snek (Autodesk Fusion 360 design; units mm, degrees)
Autodesk Fusion 360 part; units mm, degrees
sketch "Sketch1" plane through (0, 0, 0) normal (0, 1, 0) x (1, 0, 0)
  spline S0 degree 3 poles (29.3103, -75.7968) (29.3103, -75.278) (29.4828, -74.6533) (29.8072, -73.9977) knots 0 0 0 0 1 1 1 1
  spline S1 degree 3 poles (29.8072, -73.9977) (30.0802, -73.4455) (30.4104, -72.7171) (30.5406, -72.3792) knots 0 0 0 0 1 1 1 1
  spline S2 degree 3 poles (30.5406, -72.3792) (30.9121, -71.4166) (34.8067, -66.1972) (35.4505, -65.7995) knots 0 0 0 0 1 1 1 1
  spline S3 degree 3 poles (35.4505, -65.7995) (35.918, -65.5106) (35.5103, -65.1333) (33.9175, -64.3814) knots 0 0 0 0 1 1 1 1
  spline S4 degree 3 poles (33.9175, -64.3814) (30.1151, -62.5864) (30.475, -62.841) (26.8195, -59.3612) knots 0 0 0 0 1 1 1 1
  spline S5 degree 3 poles (26.8195, -59.3612) (25.1375, -57.7599) (29.2799, -57.0601) (33.624, -58.2115) knots 0 0 0 0 1 1 1 1
  spline S6 degree 3 poles (33.624, -58.2115) (37.4637, -59.2291) (41.6224, -60.9553) (44.4921, -62.7222) knots 0 0 0 0 1 1 1 1
  line L0 (44.4921, -62.7222) -> (45.7208, -63.4786)
  line L1 (45.7208, -63.4786) -> (49.1432, -63.3633)
  spline S7 degree 3 poles (49.1432, -63.3633) (58.6515, -63.0423) (60.9023, -62.6732) (60.9023, -61.435) knots 0 0 0 0 1 1 1 1
  spline S8 degree 3 poles (60.9023, -61.435) (60.9023, -60.7743) (57.5045, -58.9706) (53.1077, -57.2969) knots 0 0 0 0 1 1 1 1
  spline S9 degree 3 poles (53.1077, -57.2969) (51.2821, -56.6021) (48.1624, -55.3189) (46.1751, -54.4455) knots 0 0 0 0 1 1 1 1
  spline S10 degree 3 poles (46.1751, -54.4455) (44.1875, -53.5721) (41.6243, -52.5132) (40.4789, -52.0925) knots 0 0 0 0 1 1 1 1
  spline S11 degree 3 poles (40.4789, -52.0925) (37.0141, -50.8199) (36.5223, -50.4214) (34.6461, -47.3689) knots 0 0 0 0 1 1 1 1
  spline S12 degree 3 poles (34.6461, -47.3689) (33.9934, -46.3072) (33.0015, -44.694) (32.4419, -43.7841) knots 0 0 0 0 1 1 1 1
  spline S13 degree 3 poles (32.4419, -43.7841) (30.8578, -41.2086) (30.8017, -40.965) (30.8052, -36.6557) knots 0 0 0 0 1 1 1 1
  line L2 (30.8052, -36.6557) -> (30.8083, -32.9629)
  line L3 (30.8083, -32.9629) -> (31.595, -31.573)
  spline S14 degree 3 poles (31.595, -31.573) (34.8697, -25.789) (41.12, -23.876) (55.3739, -24.2957) knots 0 0 0 0 1 1 1 1
  spline S15 degree 3 poles (55.3739, -24.2957) (62.7089, -24.5116) (63.6588, -24.6338) (67.6595, -25.8789) knots 0 0 0 0 1 1 1 1
  spline S16 degree 3 poles (67.6595, -25.8789) (68.2387, -26.0591) (70.9941, -26.9198) (73.7822, -27.7916) knots 0 0 0 0 1 1 1 1
  spline S17 degree 3 poles (73.7822, -27.7916) (78.3857, -29.2307) (78.9387, -29.3664) (79.7965, -29.2656) knots 0 0 0 0 1 1 1 1
  spline S18 degree 3 poles (79.7965, -29.2656) (81.5671, -29.0574) (82.6505, -30.8647) (81.1967, -31.6006) knots 0 0 0 0 1 1 1 1
  spline S19 degree 3 poles (81.1967, -31.6006) (80.2539, -32.0776) (80.0513, -32.339) (80.1505, -32.9502) knots 0 0 0 0 1 1 1 1
  spline S20 degree 3 poles (80.1505, -32.9502) (80.3079, -33.9194) (79.8743, -34.1249) (77.1004, -34.3969) knots 0 0 0 0 1 1 1 1
  spline S21 degree 3 poles (77.1004, -34.3969) (75.7693, -34.5274) (74.1667, -34.7187) (73.5394, -34.8216) knots 0 0 0 0 1 1 1 1
  spline S22 degree 3 poles (73.5394, -34.8216) (72.1064, -35.0568) (68.358, -34.6904) (64.6139, -33.949) knots 0 0 0 0 1 1 1 1
  spline S23 degree 3 poles (64.6139, -33.949) (55.5281, -32.1498) (47.0855, -31.9747) (44.4304, -33.5304) knots 0 0 0 0 1 1 1 1
  spline S24 degree 3 poles (44.4304, -33.5304) (41.8722, -35.0293) (40.5109, -38.4289) (41.2446, -41.4867) knots 0 0 0 0 1 1 1 1
  spline S25 degree 3 poles (41.2446, -41.4867) (41.8722, -44.1029) (47.5835, -46.9927) (55.1236, -48.509) knots 0 0 0 0 1 1 1 1
  spline S26 degree 3 poles (55.1236, -48.509) (62.1797, -49.928) (66.012, -51.9758) (68.9787, -55.9129) knots 0 0 0 0 1 1 1 1
  spline S27 degree 3 poles (68.9787, -55.9129) (71.8979, -59.7871) (72.8025, -63.3955) (71.6878, -66.7184) knots 0 0 0 0 1 1 1 1
  spline S28 degree 3 poles (71.6878, -66.7184) (69.8733, -72.1265) (67.651, -73.1063) (58.0943, -72.7105) knots 0 0 0 0 1 1 1 1
  spline S29 degree 3 poles (58.0943, -72.7105) (54.8606, -72.5766) (50.7534, -72.4631) (48.9678, -72.4583) knots 0 0 0 0 1 1 1 1
  spline S30 degree 3 poles (48.9678, -72.4583) (46.7426, -72.4522) (45.5549, -72.3789) (45.1943, -72.2252) knots 0 0 0 0 1 1 1 1
  spline S31 degree 3 poles (45.1943, -72.2252) (44.5603, -71.9553) (41.6888, -71.3328) (41.0602, -71.3291) knots 0 0 0 0 1 1 1 1
  spline S32 degree 3 poles (41.0602, -71.3291) (40.5273, -71.3256) (39.7507, -72.0924) (39.0493, -73.3145) knots 0 0 0 0 1 1 1 1
  spline S33 degree 3 poles (39.0493, -73.3145) (37.8719, -75.3658) (36.8498, -75.8725) (36.1553, -74.7488) knots 0 0 0 0 1 1 1 1
  spline S34 degree 3 poles (36.1553, -74.7488) (35.6719, -73.9667) (35.8632, -73.9278) (33.1203, -75.3629) knots 0 0 0 0 1 1 1 1
  spline S35 degree 3 poles (33.1203, -75.3629) (31.3074, -76.3114) (30.6057, -76.5916) (30.0413, -76.5916) knots 0 0 0 0 1 1 1 1
  line L4 (30.0413, -76.5916) -> (29.3103, -76.5916)
  line L5 (29.3103, -76.5916) -> (29.3103, -75.7968)
  spline S36 degree 3 poles (35.8775, -71.6704) (35.9746, -71.5757) (35.9137, -71.237) (35.724, -70.8163) knots 0 0 0 0 1 1 1 1
  spline S37 degree 3 poles (35.724, -70.8163) (34.9062, -69.0028) (36.4964, -68.0477) (37.8584, -69.5344) knots 0 0 0 0 1 1 1 1
  line L6 (37.8584, -69.5344) -> (38.4207, -70.1485)
  line L7 (38.4207, -70.1485) -> (39.4496, -69.8598)
  spline S38 degree 3 poles (39.4496, -69.8598) (40.0153, -69.7011) (40.993, -69.5712) (41.6219, -69.5712) knots 0 0 0 0 1 1 1 1
  line L8 (41.6219, -69.5712) -> (42.7651, -69.5712)
  line L9 (42.7651, -69.5712) -> (43.3443, -68.765)
  spline S39 degree 3 poles (43.3443, -68.765) (44.886, -66.6179) (46.8313, -66.846) (47.0011, -69.1936) knots 0 0 0 0 1 1 1 1
  spline S40 degree 3 poles (47.0011, -69.1936) (47.0477, -69.836) (47.1596, -70.2718) (47.2776, -70.2697) knots 0 0 0 0 1 1 1 1
  spline S41 degree 3 poles (47.2776, -70.2697) (47.3866, -70.2678) (48.3312, -70.1525) (49.3765, -70.0133) knots 0 0 0 0 1 1 1 1
  spline S42 degree 3 poles (49.3765, -70.0133) (51.1482, -69.7775) (51.389, -69.7834) (52.9196, -70.0982) knots 0 0 0 0 1 1 1 1
  spline S43 degree 3 poles (52.9196, -70.0982) (58.5512, -71.2571) (65.4124, -70.9547) (67.6103, -69.4508) knots 0 0 0 0 1 1 1 1
  spline S44 degree 3 poles (67.6103, -69.4508) (69.6047, -68.0866) (70.5818, -64.2419) (69.6534, -61.4135) knots 0 0 0 0 1 1 1 1
  spline S45 degree 3 poles (69.6534, -61.4135) (69.1793, -59.97) (68.9761, -59.9623) (68.9761, -61.3884) knots 0 0 0 0 1 1 1 1
  spline S46 degree 3 poles (68.9761, -61.3884) (68.9761, -63.984) (67.8765, -63.2474) (67.5674, -60.4446) knots 0 0 0 0 1 1 1 1
  spline S47 degree 3 poles (67.5674, -60.4446) (67.1227, -56.41) (65.7439, -54.6108) (61.5167, -52.5487) knots 0 0 0 0 1 1 1 1
  spline S48 degree 3 poles (61.5167, -52.5487) (59.1042, -51.3715) (57.6249, -50.9683) (52.1269, -49.9891) knots 0 0 0 0 1 1 1 1
  spline S49 degree 3 poles (52.1269, -49.9891) (48.1394, -49.2787) (43.8092, -47.3393) (41.1242, -45.0615) knots 0 0 0 0 1 1 1 1
  spline S50 degree 3 poles (41.1242, -45.0615) (38.7247, -43.0253) (38.2204, -37.7807) (40.15, -34.9258) knots 0 0 0 0 1 1 1 1
  spline S51 degree 3 poles (40.15, -34.9258) (42.8884, -30.8745) (45.8338, -29.9183) (54.1451, -30.3821) knots 0 0 0 0 1 1 1 1
  spline S52 degree 3 poles (54.1451, -30.3821) (56.6883, -30.524) (57.2132, -30.5094) (57.6987, -30.2827) knots 0 0 0 0 1 1 1 1
  spline S53 degree 3 poles (57.6987, -30.2827) (58.2433, -30.0284) (58.3681, -30.0493) (60.507, -30.7544) knots 0 0 0 0 1 1 1 1
  spline S54 degree 3 poles (60.507, -30.7544) (65.0624, -32.2559) (68.6115, -32.6917) (73.7153, -32.3763) knots 0 0 0 0 1 1 1 1
  spline S55 degree 3 poles (73.7153, -32.3763) (79.2983, -32.0313) (79.2578, -31.6887) (73.4076, -29.7633) knots 0 0 0 0 1 1 1 1
  spline S56 degree 3 poles (73.4076, -29.7633) (64.7663, -26.9195) (60.4938, -26.2258) (51.6004, -26.2221) knots 0 0 0 0 1 1 1 1
  spline S57 degree 3 poles (51.6004, -26.2221) (42.1579, -26.2184) (35.3579, -28.4938) (33.4277, -32.3028) knots 0 0 0 0 1 1 1 1
  line L10 (33.4277, -32.3028) -> (32.9083, -33.328)
  line L11 (32.9083, -33.328) -> (32.9083, -36.7504)
  line L12 (32.9083, -36.7504) -> (32.9083, -40.1731)
  line L13 (32.9083, -40.1731) -> (33.4518, -41.3137)
  spline S58 degree 3 poles (33.4518, -41.3137) (33.7505, -41.9413) (34.4218, -43.0475) (34.9435, -43.7724) knots 0 0 0 0 1 1 1 1
  spline S59 degree 3 poles (34.9435, -43.7724) (35.4653, -44.4971) (36.1984, -45.6817) (36.5731, -46.405) knots 0 0 0 0 1 1 1 1
  spline S60 degree 3 poles (36.5731, -46.405) (37.7756, -48.7265) (38.3421, -49.135) (42.4519, -50.645) knots 0 0 0 0 1 1 1 1
  spline S61 degree 3 poles (42.4519, -50.645) (45.7589, -51.86) (48.2669, -52.8995) (49.9914, -53.77) knots 0 0 0 0 1 1 1 1
  spline S62 degree 3 poles (49.9914, -53.77) (50.7958, -54.1761) (53.0701, -55.1244) (55.0455, -55.8774) knots 0 0 0 0 1 1 1 1
  spline S63 degree 3 poles (55.0455, -55.8774) (58.5708, -57.2212) (59.5307, -57.7237) (61.3947, -59.2027) knots 0 0 0 0 1 1 1 1
  spline S64 degree 3 poles (61.3947, -59.2027) (64.5139, -61.6773) (62.9571, -64.247) (57.8625, -65.0338) knots 0 0 0 0 1 1 1 1
  spline S65 degree 3 poles (57.8625, -65.0338) (52.8259, -65.8117) (43.7023, -65.6844) (43.7023, -64.8362) knots 0 0 0 0 1 1 1 1
  spline S66 degree 3 poles (43.7023, -64.8362) (43.7023, -64.3441) (41.7303, -63.3815) (36.4577, -61.2998) knots 0 0 0 0 1 1 1 1
  spline S67 degree 3 poles (36.4577, -61.2998) (33.8217, -60.2592) (30.7144, -59.5847) (30.7144, -60.0531) knots 0 0 0 0 1 1 1 1
  spline S68 degree 3 poles (30.7144, -60.0531) (30.7144, -60.3629) (31.4399, -60.7976) (36.241, -63.3635) knots 0 0 0 0 1 1 1 1
  spline S69 degree 3 poles (36.241, -63.3635) (39.0403, -64.8597) (39.1933, -65.4757) (37.1991, -67.2246) knots 0 0 0 0 1 1 1 1
  spline S70 degree 3 poles (37.1991, -67.2246) (35.5653, -68.6576) (32.4697, -72.4226) (32.4697, -72.9769) knots 0 0 0 0 1 1 1 1
  spline S71 degree 3 poles (32.4697, -72.9769) (32.4697, -73.2227) (35.4616, -72.0757) (35.8775, -71.6704) knots 0 0 0 0 1 1 1 1
  spline S72 degree 3 poles (53.1799, -52.9781) (51.7803, -52.3428) (50.5357, -51.7795) (50.4142, -51.7266) knots 0 0 0 0 1 1 1 1
  spline S73 degree 3 poles (50.4142, -51.7266) (50.1637, -51.6173) (49.9218, -50.8318) (50.0875, -50.6662) knots 0 0 0 0 1 1 1 1
  spline S74 degree 3 poles (50.0875, -50.6662) (50.4153, -50.3383) (57.0373, -52.8074) (57.0405, -53.2588) knots 0 0 0 0 1 1 1 1
  spline S75 degree 3 poles (57.0405, -53.2588) (57.0479, -54.3134) (55.9446, -54.2333) (53.1799, -52.9781) knots 0 0 0 0 1 1 1 1
  spline S76 degree 3 poles (36.7927, -44.7416) (36.1196, -43.5909) (36.0751, -43.1486) (36.5898, -42.7215) knots 0 0 0 0 1 1 1 1
  spline S77 degree 3 poles (36.5898, -42.7215) (36.98, -42.3977) (37.4711, -42.7792) (37.9809, -43.8023) knots 0 0 0 0 1 1 1 1
  spline S78 degree 3 poles (37.9809, -43.8023) (39.0805, -46.009) (38.023, -46.8448) (36.7927, -44.7416) knots 0 0 0 0 1 1 1 1
  line L14 (36.3667, -33.7172) -> (35.9905, -33.3169)
  line L15 (35.9905, -33.3169) -> (37.1369, -31.304)
  spline S79 degree 3 poles (37.1369, -31.304) (38.8284, -28.3345) (38.7146, -28.4756) (39.2279, -28.7095) knots 0 0 0 0 1 1 1 1
  spline S80 degree 3 poles (39.2279, -28.7095) (39.842, -28.9891) (39.7925, -29.2431) (38.6853, -31.5032) knots 0 0 0 0 1 1 1 1
  spline S81 degree 3 poles (38.6853, -31.5032) (37.3351, -34.2588) (37.093, -34.4903) (36.3667, -33.7172) knots 0 0 0 0 1 1 1 1
  spline S82 degree 3 poles (59.5148, -29.577) (58.9246, -29.4117) (58.6655, -28.9582) (58.9595, -28.6039) knots 0 0 0 0 1 1 1 1
  spline S83 degree 3 poles (58.9595, -28.6039) (59.3233, -28.1657) (61.277, -28.2181) (61.6921, -28.6769) knots 0 0 0 0 1 1 1 1
  spline S84 degree 3 poles (61.6921, -28.6769) (62.3798, -29.4365) (61.0206, -29.9982) (59.5148, -29.577) knots 0 0 0 0 1 1 1 1
  spline S85 degree 3 poles (93.6588, -25.1336) (93.2897, -24.5624) (93.1757, -14.4698) (93.5334, -14.0388) knots 0 0 0 0 1 1 1 1
  spline S86 degree 3 poles (93.5334, -14.0388) (94.2075, -13.2266) (94.9516, -13.9973) (94.9516, -15.5081) knots 0 0 0 0 1 1 1 1
  spline S87 degree 3 poles (94.9516, -15.5081) (94.9516, -16.5563) (95.1876, -17.0643) (95.6852, -17.0876) knots 0 0 0 0 1 1 1 1
  spline S88 degree 3 poles (95.6852, -17.0876) (95.8477, -17.0953) (96.7975, -15.6692) (97.3299, -14.6183) knots 0 0 0 0 1 1 1 1
  spline S89 degree 3 poles (97.3299, -14.6183) (97.836, -13.6195) (98.43, -13.4546) (98.906, -14.1806) knots 0 0 0 0 1 1 1 1
  spline S90 degree 3 poles (98.906, -14.1806) (99.2468, -14.7008) (99.0595, -15.2273) (97.8358, -17.1911) knots 0 0 0 0 1 1 1 1
  line L16 (97.8358, -17.1911) -> (97.0304, -18.483)
  line L17 (97.0304, -18.483) -> (97.9215, -19.5845)
  spline S91 degree 3 poles (97.9215, -19.5845) (98.9097, -20.8061) (99.0581, -21.4649) (98.4417, -21.8967) knots 0 0 0 0 1 1 1 1
  spline S92 degree 3 poles (98.4417, -21.8967) (97.9234, -22.2597) (97.7506, -22.1515) (96.4189, -20.6307) knots 0 0 0 0 1 1 1 1
  spline S93 degree 3 poles (96.4189, -20.6307) (95.7718, -19.8917) (95.204, -19.307) (95.1571, -19.3313) knots 0 0 0 0 1 1 1 1
  spline S94 degree 3 poles (95.1571, -19.3313) (95.11, -19.3556) (95.0857, -20.5404) (95.1029, -21.9642) knots 0 0 0 0 1 1 1 1
  spline S95 degree 3 poles (95.1029, -21.9642) (95.1365, -24.7521) (94.992, -25.385) (94.3001, -25.4847) knots 0 0 0 0 1 1 1 1
  spline S96 degree 3 poles (94.3001, -25.4847) (94.0562, -25.5199) (93.8271, -25.3945) (93.6588, -25.1336) knots 0 0 0 0 1 1 1 1
  spline S97 degree 3 poles (34.7869, -23.8382) (34.4689, -23.6154) (34.4003, -23.3977) (34.4003, -22.6119) knots 0 0 0 0 1 1 1 1
  line L18 (34.4003, -22.6119) -> (34.4003, -21.6565)
  line L19 (34.4003, -21.6565) -> (33.7045, -21.6565)
  spline S98 degree 3 poles (33.7045, -21.6565) (32.97, -21.6565) (32.6451, -21.34) (32.6451, -20.6248) knots 0 0 0 0 1 1 1 1
  spline S99 degree 3 poles (32.6451, -20.6248) (32.6451, -20.1819) (33.2788, -19.7258) (33.8939, -19.7258) knots 0 0 0 0 1 1 1 1
  spline S100 degree 3 poles (33.8939, -19.7258) (34.5361, -19.7258) (34.5757, -19.5427) (34.5757, -16.5873) knots 0 0 0 0 1 1 1 1
  spline S101 degree 3 poles (34.5757, -16.5873) (34.5757, -13.8557) (34.6501, -13.583) (35.3944, -13.583) knots 0 0 0 0 1 1 1 1
  spline S102 degree 3 poles (35.3944, -13.583) (36.0931, -13.583) (36.2212, -14.1478) (36.1778, -17.0389) knots 0 0 0 0 1 1 1 1
  line L20 (36.1778, -17.0389) -> (36.1381, -19.7049)
  line L21 (36.1381, -19.7049) -> (36.8872, -19.7591)
  spline S103 degree 3 poles (36.8872, -19.7591) (38.4723, -19.8745) (38.5302, -21.6565) (36.9488, -21.6565) knots 0 0 0 0 1 1 1 1
  spline S104 degree 3 poles (36.9488, -21.6565) (36.1741, -21.6565) (36.155, -21.6699) (36.1378, -22.2269) knots 0 0 0 0 1 1 1 1
  spline S105 degree 3 poles (36.1378, -22.2269) (36.095, -23.6236) (35.4978, -24.3359) (34.7869, -23.8382) knots 0 0 0 0 1 1 1 1
  spline S106 degree 3 poles (9.8192, -21.5572) (9.5142, -21.1897) (9.3625, -14.4767) (9.6475, -13.9446) knots 0 0 0 0 1 1 1 1
  spline S107 degree 3 poles (9.6475, -13.9446) (10.2545, -12.8104) (11.2326, -13.8372) (11.2326, -15.6091) knots 0 0 0 0 1 1 1 1
  spline S108 degree 3 poles (11.2326, -15.6091) (11.2326, -17.0067) (11.598, -18.3044) (12.2306, -19.1553) knots 0 0 0 0 1 1 1 1
  spline S109 degree 3 poles (12.2306, -19.1553) (12.9987, -20.1885) (13.1032, -19.9729) (13.2083, -17.1371) knots 0 0 0 0 1 1 1 1
  spline S110 degree 3 poles (13.2083, -17.1371) (13.322, -14.0761) (13.4604, -13.583) (14.206, -13.583) knots 0 0 0 0 1 1 1 1
  spline S111 degree 3 poles (14.206, -13.583) (14.5386, -13.583) (14.7947, -13.7031) (14.9061, -13.911) knots 0 0 0 0 1 1 1 1
  spline S112 degree 3 poles (14.9061, -13.911) (15.1162, -14.3032) (14.8421, -19.7933) (14.578, -20.4881) knots 0 0 0 0 1 1 1 1
  spline S113 degree 3 poles (14.578, -20.4881) (14.1097, -21.7197) (12.7876, -22.0562) (11.7726, -21.2022) knots 0 0 0 0 1 1 1 1
  spline S114 degree 3 poles (11.7726, -21.2022) (11.3726, -20.8653) (11.2326, -20.8167) (11.2326, -21.014) knots 0 0 0 0 1 1 1 1
  spline S115 degree 3 poles (11.2326, -21.014) (11.2326, -21.6972) (10.2492, -22.0753) (9.8192, -21.5572) knots 0 0 0 0 1 1 1 1
  spline S116 degree 3 poles (45.5663, -21.4578) (45.2572, -21.0164) (45.3604, -10.518) (45.6779, -10.1167) knots 0 0 0 0 1 1 1 1
  spline S117 degree 3 poles (45.6779, -10.1167) (46.4069, -9.1951) (47.0371, -10.1278) (47.0371, -12.128) knots 0 0 0 0 1 1 1 1
  line L22 (47.0371, -12.128) -> (47.0371, -13.6801)
  line L23 (47.0371, -13.6801) -> (47.7343, -13.6137)
  spline S118 degree 3 poles (47.7343, -13.6137) (50.3301, -13.366) (51.8594, -17.0916) (50.3997, -20.1071) knots 0 0 0 0 1 1 1 1
  spline S119 degree 3 poles (50.3997, -20.1071) (49.7933, -21.3596) (48.1907, -21.8647) (47.2607, -21.0963) knots 0 0 0 0 1 1 1 1
  spline S120 degree 3 poles (47.2607, -21.0963) (47.1048, -20.9675) (46.9887, -21.0442) (46.8376, -21.3755) knots 0 0 0 0 1 1 1 1
  spline S121 degree 3 poles (46.8376, -21.3755) (46.5796, -21.9419) (45.9346, -21.9837) (45.5663, -21.4578) knots 0 0 0 0 1 1 1 1
  spline S122 degree 3 poles (63.3997, -21.6125) (63.3016, -21.4919) (63.1661, -19.8531) (63.0986, -17.9708) knots 0 0 0 0 1 1 1 1
  spline S123 degree 3 poles (63.0986, -17.9708) (62.9584, -14.0555) (63.042, -13.583) (63.8757, -13.583) knots 0 0 0 0 1 1 1 1
  spline S124 degree 3 poles (63.8757, -13.583) (64.5745, -13.583) (64.6933, -13.8677) (64.8277, -15.8647) knots 0 0 0 0 1 1 1 1
  spline S125 degree 3 poles (64.8277, -15.8647) (64.9454, -17.6142) (65.5349, -19.2244) (66.2032, -19.6231) knots 0 0 0 0 1 1 1 1
  spline S126 degree 3 poles (66.2032, -19.6231) (66.6713, -19.9023) (66.7139, -19.7298) (66.7697, -17.3305) knots 0 0 0 0 1 1 1 1
  spline S127 degree 3 poles (66.7697, -17.3305) (66.838, -14.4127) (67.051, -13.583) (67.7325, -13.583) knots 0 0 0 0 1 1 1 1
  spline S128 degree 3 poles (67.7325, -13.583) (68.611, -13.583) (68.6554, -13.7912) (68.4723, -17.0442) knots 0 0 0 0 1 1 1 1
  spline S129 degree 3 poles (68.4723, -17.0442) (68.2942, -20.2049) (68.0704, -21.1201) (67.3859, -21.4866) knots 0 0 0 0 1 1 1 1
  spline S130 degree 3 poles (67.3859, -21.4866) (66.8531, -21.7718) (65.6926, -21.5906) (65.2222, -21.1485) knots 0 0 0 0 1 1 1 1
  line L24 (65.2222, -21.1485) -> (64.8375, -20.787)
  line L25 (64.8375, -20.787) -> (64.6404, -21.3096)
  spline S131 degree 3 poles (64.6404, -21.3096) (64.4282, -21.8718) (63.7458, -22.0385) (63.3997, -21.6125) knots 0 0 0 0 1 1 1 1
  spline S132 degree 3 poles (80.5873, -21.6019) (80.2587, -21.2061) (80.2333, -13.9648) (80.5598, -13.7565) knots 0 0 0 0 1 1 1 1
  spline S133 degree 3 poles (80.5598, -13.7565) (81.5187, -13.1443) (81.883, -13.6565) (82.0153, -15.8028) knots 0 0 0 0 1 1 1 1
  spline S134 degree 3 poles (82.0153, -15.8028) (82.1542, -18.0592) (83.0276, -19.9615) (83.7898, -19.6689) knots 0 0 0 0 1 1 1 1
  spline S135 degree 3 poles (83.7898, -19.6689) (83.9952, -19.5901) (84.0298, -19.3382) (83.9565, -18.4629) knots 0 0 0 0 1 1 1 1
  spline S136 degree 3 poles (83.9565, -18.4629) (83.6816, -15.1763) (84.6182, -12.6037) (85.6411, -13.8359) knots 0 0 0 0 1 1 1 1
  spline S137 degree 3 poles (85.6411, -13.8359) (85.9547, -14.214) (85.5906, -20.0443) (85.2069, -20.7862) knots 0 0 0 0 1 1 1 1
  spline S138 degree 3 poles (85.2069, -20.7862) (84.6624, -21.839) (83.2556, -21.9615) (82.324, -21.0371) knots 0 0 0 0 1 1 1 1
  spline S139 degree 3 poles (82.324, -21.0371) (82.1029, -20.8175) (82.0415, -20.8526) (81.8499, -21.3085) knots 0 0 0 0 1 1 1 1
  spline S140 degree 3 poles (81.8499, -21.3085) (81.611, -21.8766) (80.944, -22.0316) (80.5873, -21.6019) knots 0 0 0 0 1 1 1 1
  spline S141 degree 3 poles (28.9491, -21.49) (26.506, -20.7487) (26.6425, -18.4949) (29.2222, -16.986) knots 0 0 0 0 1 1 1 1
  spline S142 degree 3 poles (29.2222, -16.986) (31.0197, -15.9343) (30.5263, -14.9921) (28.5107, -15.6277) knots 0 0 0 0 1 1 1 1
  spline S143 degree 3 poles (28.5107, -15.6277) (27.4548, -15.9605) (27.0288, -15.801) (27.0288, -15.0728) knots 0 0 0 0 1 1 1 1
  spline S144 degree 3 poles (27.0288, -15.0728) (27.0288, -13.2181) (30.9906, -13.1022) (31.8587, -14.9315) knots 0 0 0 0 1 1 1 1
  spline S145 degree 3 poles (31.8587, -14.9315) (32.5051, -16.2936) (32.0664, -17.1927) (30.144, -18.4447) knots 0 0 0 0 1 1 1 1
  spline S146 degree 3 poles (30.144, -18.4447) (28.9044, -19.2522) (28.6925, -19.6133) (29.3542, -19.7909) knots 0 0 0 0 1 1 1 1
  spline S147 degree 3 poles (29.3542, -19.7909) (30.0953, -19.9893) (30.5702, -19.9017) (30.8949, -19.5064) knots 0 0 0 0 1 1 1 1
  spline S148 degree 3 poles (30.8949, -19.5064) (31.3947, -18.8979) (31.8405, -19.2691) (31.9103, -20.3523) knots 0 0 0 0 1 1 1 1
  spline S149 degree 3 poles (31.9103, -20.3523) (31.9894, -21.5787) (30.7766, -22.0446) (28.9491, -21.49) knots 0 0 0 0 1 1 1 1
  spline S150 degree 3 poles (76.0547, -21.4638) (73.8926, -20.8378) (74.1143, -18.4317) (76.4646, -17.0183) knots 0 0 0 0 1 1 1 1
  spline S151 degree 3 poles (76.4646, -17.0183) (78.3278, -15.8978) (77.9687, -14.995) (75.8992, -15.5967) knots 0 0 0 0 1 1 1 1
  spline S152 degree 3 poles (75.8992, -15.5967) (74.5855, -15.9785) (74.0555, -15.6737) (74.4106, -14.74) knots 0 0 0 0 1 1 1 1
  spline S153 degree 3 poles (74.4106, -14.74) (74.8916, -13.475) (77.348, -13.1869) (78.6098, -14.2476) knots 0 0 0 0 1 1 1 1
  spline S154 degree 3 poles (78.6098, -14.2476) (80.0346, -15.4454) (79.5819, -17.1104) (77.4745, -18.4238) knots 0 0 0 0 1 1 1 1
  spline S155 degree 3 poles (77.4745, -18.4238) (76.0857, -19.2895) (75.978, -19.4342) (76.5114, -19.7197) knots 0 0 0 0 1 1 1 1
  spline S156 degree 3 poles (76.5114, -19.7197) (77.0565, -20.0115) (77.8227, -19.9322) (78.1495, -19.5504) knots 0 0 0 0 1 1 1 1
  spline S157 degree 3 poles (78.1495, -19.5504) (78.972, -18.5897) (79.8161, -20.184) (79.058, -21.2665) knots 0 0 0 0 1 1 1 1
  spline S158 degree 3 poles (79.058, -21.2665) (78.7575, -21.6956) (77.207, -21.7975) (76.0547, -21.4638) knots 0 0 0 0 1 1 1 1
  spline S159 degree 3 poles (17.6302, -21.2342) (16.4042, -20.7) (15.5898, -19.1731) (15.5623, -17.3564) knots 0 0 0 0 1 1 1 1
  spline S160 degree 3 poles (15.5623, -17.3564) (15.4956, -12.9215) (20.1753, -12.2103) (21.0698, -16.5196) knots 0 0 0 0 1 1 1 1
  spline S161 degree 3 poles (21.0698, -16.5196) (21.7276, -19.6882) (19.8837, -22.2155) (17.6302, -21.2342) knots 0 0 0 0 1 1 1 1
  spline S162 degree 3 poles (40.5432, -21.3577) (38.1262, -20.4814) (37.6933, -15.4075) (39.9288, -14.1571) knots 0 0 0 0 1 1 1 1
  spline S163 degree 3 poles (39.9288, -14.1571) (41.6846, -13.175) (44.59, -14.0849) (44.3714, -15.5485) knots 0 0 0 0 1 1 1 1
  spline S164 degree 3 poles (44.3714, -15.5485) (44.2727, -16.2105) (43.7997, -16.3349) (43.0292, -15.902) knots 0 0 0 0 1 1 1 1
  spline S165 degree 3 poles (43.0292, -15.902) (42.1741, -15.4213) (41.0808, -15.3938) (40.531, -15.8393) knots 0 0 0 0 1 1 1 1
  line L26 (40.531, -15.8393) -> (40.1288, -16.1648)
  line L27 (40.1288, -16.1648) -> (41.6729, -17.0239)
  spline S166 degree 3 poles (41.6729, -17.0239) (43.9605, -18.2965) (44.6035, -19.389) (43.7671, -20.583) knots 0 0 0 0 1 1 1 1
  spline S167 degree 3 poles (43.7671, -20.583) (43.2604, -21.3061) (41.5409, -21.7194) (40.5432, -21.3577) knots 0 0 0 0 1 1 1 1
  spline S168 degree 3 poles (58.7087, -21.2323) (57.4003, -20.6484) (56.6415, -19.2239) (56.6356, -17.3406) knots 0 0 0 0 1 1 1 1
  spline S169 degree 3 poles (56.6356, -17.3406) (56.6214, -12.8786) (61.2418, -12.1955) (62.1408, -16.5264) knots 0 0 0 0 1 1 1 1
  spline S170 degree 3 poles (62.1408, -16.5264) (62.7991, -19.6972) (60.9497, -22.2327) (58.7087, -21.2323) knots 0 0 0 0 1 1 1 1
  spline S171 degree 3 poles (88.37, -21.2768) (86.0729, -20.0094) (85.5988, -15.6959) (87.5996, -14.2711) knots 0 0 0 0 1 1 1 1
  spline S172 degree 3 poles (87.5996, -14.2711) (89.1921, -13.1371) (92.3189, -13.9386) (92.3189, -15.4806) knots 0 0 0 0 1 1 1 1
  spline S173 degree 3 poles (92.3189, -15.4806) (92.3189, -16.1669) (91.849, -16.3132) (90.9876, -15.8946) knots 0 0 0 0 1 1 1 1
  spline S174 degree 3 poles (90.9876, -15.8946) (90.0242, -15.4266) (88.9857, -15.4017) (88.4518, -15.8343) knots 0 0 0 0 1 1 1 1
  line L28 (88.4518, -15.8343) -> (88.0557, -16.1547)
  line L29 (88.0557, -16.1547) -> (89.5937, -17.018)
  spline S175 degree 3 poles (89.5937, -17.018) (91.8766, -18.2994) (92.5163, -19.3916) (91.6818, -20.583) knots 0 0 0 0 1 1 1 1
  spline S176 degree 3 poles (91.6818, -20.583) (91.1323, -21.3675) (89.2495, -21.762) (88.37, -21.2768) knots 0 0 0 0 1 1 1 1
  spline S177 degree 3 poles (90.3065, -19.5408) (90.4079, -19.3765) (88.138, -18.0565) (87.997, -18.1976) knots 0 0 0 0 1 1 1 1
  spline S178 degree 3 poles (87.997, -18.1976) (87.8517, -18.3425) (88.4203, -19.3289) (88.8042, -19.5977) knots 0 0 0 0 1 1 1 1
  spline S179 degree 3 poles (88.8042, -19.5977) (89.1569, -19.8448) (90.1417, -19.8075) (90.3065, -19.5408) knots 0 0 0 0 1 1 1 1
  spline S180 degree 3 poles (42.2682, -19.5726) (42.4381, -19.4649) (42.2944, -19.3046) (41.7417, -18.985) knots 0 0 0 0 1 1 1 1
  spline S181 degree 3 poles (41.7417, -18.985) (40.231, -18.111) (40.1921, -18.0981) (40.1921, -18.4656) knots 0 0 0 0 1 1 1 1
  spline S182 degree 3 poles (40.1921, -18.4656) (40.1921, -19.3083) (41.5462, -20.0303) (42.2682, -19.5726) knots 0 0 0 0 1 1 1 1
  spline S183 degree 3 poles (19.2072, -19.2117) (19.6853, -18.6836) (19.6813, -16.7466) (19.2011, -16.0984) knots 0 0 0 0 1 1 1 1
  spline S184 degree 3 poles (19.2011, -16.0984) (18.3954, -15.0112) (17.2, -15.6652) (17.2, -17.1932) knots 0 0 0 0 1 1 1 1
  spline S185 degree 3 poles (17.2, -17.1932) (17.2, -18.9635) (18.3684, -20.1385) (19.2072, -19.2117) knots 0 0 0 0 1 1 1 1
  spline S186 degree 3 poles (48.855, -19.3271) (50.1031, -18.4145) (49.0903, -15.3199) (47.6329, -15.5933) knots 0 0 0 0 1 1 1 1
  line L30 (47.6329, -15.5933) -> (47.0371, -15.7049)
  line L31 (47.0371, -15.7049) -> (47.0371, -17.2593)
  line L32 (47.0371, -17.2593) -> (47.0371, -18.8138)
  line L33 (47.0371, -18.8138) -> (47.6075, -19.1792)
  spline S187 degree 3 poles (47.6075, -19.1792) (48.2761, -19.6073) (48.4444, -19.6274) (48.855, -19.3271) knots 0 0 0 0 1 1 1 1
  spline S188 degree 3 poles (60.2885, -19.199) (60.7724, -18.6643) (60.7613, -16.7595) (60.2708, -16.0981) knots 0 0 0 0 1 1 1 1
  spline S189 degree 3 poles (60.2708, -16.0981) (59.4595, -15.0043) (58.2697, -15.6655) (58.2697, -17.2104) knots 0 0 0 0 1 1 1 1
  spline S190 degree 3 poles (58.2697, -17.2104) (58.2697, -19.0043) (59.4302, -20.1473) (60.2885, -19.199) knots 0 0 0 0 1 1 1 1
extrude "Extrude1" add sketch "Sketch1" against normal blind 2 makes body 1 at (85.0699, 0, 16.8883) makes body 2 at (46.0258, 0, 14.2872) makes body 3 at (20.6044, 0, 17.0987) makes body 4 at (38.0899, -0.8889, 44.0319) makes body 5 at (53.2482, -0.8889, 51.5096) makes body 6 at (10.301, 0, 18.7504) makes body 7 at (39.6163, 0, 17.1921) makes body 8 at (76.656, 0, 18.2774) makes body 9 at (87.4644, 0, 17.1592) makes body 10 at (61.6781, 0, 17.0975) makes body 11 at (29.4022, 0, 18.2614) makes body 12 at (36.9243, 0, 32.6982) makes body 13 at (60.3513, 0, 32.4662) makes body 14 at (59.7641, -1.1111, 29.6383) makes body 15 at (35.6253, 0, 18.3522) makes body 16 at (63.6723, 0, 16.1218) makes body 17 at (94.0055, 0, 22.1582)
sketch "Sketch2" plane through (0, 0, 0) normal (0, 1, 0) x (1, 0, 0)
  line L0 (102.0389, -79.7068) -> (6.0389, -79.7068)
  line L1 (6.0389, -79.7068) -> (6.0389, -7.7068)
  line L2 (6.0389, -7.7068) -> (102.0389, -7.7068)
  line L3 (102.0389, -7.7068) -> (102.0389, -79.7068)
  dimension "d6" = 96
  dimension "d7" = 72
  constraint horizontal L0
  constraint vertical L1
  constraint horizontal L2
  constraint vertical L3
  measures "d6" distance of L0.start L0.end
  measures "d7" distance of L0.start L2.end
extrude "Extrude2" add sketch "Sketch2" along normal blind 2 bodies 1 2 3 4 5 6 7 8 9 10 11 12 13 14 15 16 17
